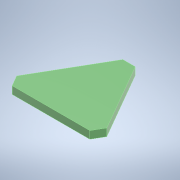
# Autodesk Inventor part: FactionSpecial_Council_CommandToken_Single
Saved by Autodesk Inventor 2021 (Build 250183000, 183)
## iProperties
Created: 2023-03-16
Part Number: FactionSpecial_Council_CommandToken_Single
Material: ABS Plastic
Document SubType Name: Modeling
Designer: Bradley
Density: 1.06 g/cm^3
Appearance: Smooth - Dark Forest Green
CouncilTriangleHeight: 22.300 mm
CouncilTriangleTrimmed: 19.600 mm
Author: Bradley
Autodesk Inventor part; units mm, degrees
ref_plane "YZ Plane" through (0, 0, 0) normal (1, 0, 0) x (0, 1, 0)
ref_plane "XZ Plane" through (0, 0, 0) normal (0, 1, 0) x (-1, 0, 0)
ref_plane "XY Plane" through (0, 0, 0) normal (0, 0, 1) x (1, 0, 0)
sketch "Sketch1" plane through (0, 0, 0) normal (0, 1, 0) x (-1, 0, 0)
  line L0 (1.5588, -12.1667) -> (-1.5588, -12.1667)
  line L1 (-1.5588, -12.1667) -> (-11.3161, 4.7333)
  line L2 (-11.3161, 4.7333) -> (-9.7572, 7.4333)
  line L3 (-9.7572, 7.4333) -> (9.7572, 7.4333)
  line L4 (9.7572, 7.4333) -> (11.3161, 4.7333)
  line L5 (11.3161, 4.7333) -> (1.5588, -12.1667)
  circle A0 centre (0, 0) radius 7.4333 construction
  line L6 (-1.5588, -12.1667) -> (-3.1177, -14.8667) construction
  line L7 (-3.1177, -14.8667) -> (-22.6321, -14.8667) construction
  line L8 (-22.6321, -14.8667) -> (-24.191, -12.1667) construction
  line L9 (-24.191, -12.1667) -> (-14.4338, 4.7333) construction
  line L10 (-14.4338, 4.7333) -> (-11.3161, 4.7333) construction
  dimension "d0" = 19.6
  dimension "d1" = 3.1177
  dimension "d4" = 14.8667
  dimension "d5" = 22.3
  constraints: 22 end point, 9 equal length, 5 parallel, 3 tangent, 2 horizontal, 1 centre point, 1 coincident
  measures "d0" distance between parallel lines of L2 L5
  measures "d1" distance of L0.start L0.end
  measures "d4" diameter of A0
  measures "d5" distance between parallel lines of L3 L7
extrude "Extrusion1" add sketch "Sketch1" along normal mid plane 1.9
equation "\"d0\" = CouncilTriangleTrimmed"
equation "\"d5\" = CouncilTriangleHeight"
equation "\"CouncilTriangleHeight\" = 22.3"
equation "\"CouncilTriangleTrimmed\" = 19.6"
body "Solid1"
